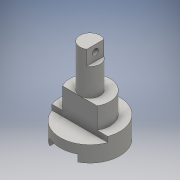
# Autodesk Inventor part: 240628_final4
Saved by Autodesk Inventor 2016 (Build 200138000, 138)
## iProperties
Created: 2024-06-28
Part Number: 240628_final4
Material: 일반
Document SubType Name: Modeling
Designer: pc
Density: 1 g/cm^3
Appearance: 기본값
Author: pc
Autodesk Inventor part; units mm, degrees
ref_plane "YZ Plane" through (0, 0, 0) normal (1, 0, 0) x (0, 1, 0)
ref_plane "XZ Plane" through (0, 0, 0) normal (0, 1, 0) x (-1, 0, 0)
ref_plane "XY Plane" through (0, 0, 0) normal (0, 0, 1) x (1, 0, 0)
sketch "스케치1" plane through (0, 0, 0) normal (0, 0, 1) x (1, 0, 0)
  circle A0 centre (0, 0) radius 14.0239
  constraints: 1 centre point, 1 coincident
extrude "돌출1" add sketch "스케치1" along normal blind 10
sketch "스케치2" plane through (0, 0, 10) normal (0, 0, 1) x (1, 0, 0)
  circle A0 centre (0, 0) radius 9.454
  constraints: 1 centre point, 1 coincident
extrude "돌출2" add sketch "스케치2" along normal blind 10
sketch "스케치3" plane through (0, 0, 20) normal (0, 0, 1) x (1, 0, 0)
  circle A0 centre (0, 0) radius 4.783
  constraints: 1 centre point, 1 coincident
extrude "돌출3" add sketch "스케치3" along normal blind 20
sketch "스케치4" plane through (0, 0, 40) normal (0, 0, 1) x (1, 0, 0)
  circle A0 centre (0, 0) radius 4.783 projected
  line L0 (7.0161, -4.0466) -> (2.5499, -4.0466)
  line L1 (2.5499, -4.0466) -> (2.5499, 4.0466)
  line L2 (2.5499, 4.0466) -> (7.0161, 4.0466)
  line L3 (7.0161, 4.0466) -> (7.0161, -4.0466)
  circle A1 centre (0, 0) radius 4.783 projected
  line L4 (7.0161, -4.0466) -> (2.5499, 4.0466) construction
  line L5 (2.5499, -4.0466) -> (7.0161, 4.0466) construction
  point P0 (4.783, 0)
  constraints: 12 end point, 2 midpoint, 2 parallel, 1 horizontal, 1 horizontal alignment, 1 perpendicular, 3 other
extrude "돌출4" cut sketch "스케치4" against normal blind 7 contours A0 L1 | A0 L2 L3 L0 picked at (3.2943, 0)
sketch "스케치5" plane through (2.5499, -4.0466, 40) normal (1, 0, 0) x (0, 0, -1)
  circle A0 centre (3.1932, 4.0466) radius 1.4587
  point P0 (40, 4.0466)
  constraints: 1 centre point
extrude "돌출5" cut sketch "스케치5" against normal blind 7
sketch "스케치6" plane through (0, 0, 20) normal (0, 0, 1) x (1, 0, 0)
  circle A0 centre (0, 0) radius 14.0239 projected
  line L0 (13.1762, -23.246) -> (-13.1762, -23.246)
  line L1 (-13.1762, -23.246) -> (-13.1762, -4.8019)
  line L2 (-13.1762, -4.8019) -> (13.1762, -4.8019)
  line L3 (13.1762, -4.8019) -> (13.1762, -23.246)
  line L4 (13.1762, -23.246) -> (-13.1762, -4.8019) construction
  line L5 (-13.1762, -23.246) -> (13.1762, -4.8019) construction
  point P0 (0, -14.0239)
  constraints: 12 end point, 2 midpoint, 2 parallel, 2 point on circle, 1 horizontal, 1 perpendicular
extrude "돌출6" cut sketch "스케치6" against normal blind 12.5 contours L2 A0 | A0 L3 L0 L1 picked at (-1.1305, -9.7665)
sketch "스케치7" plane through (0, 0, 0) normal (0, 0, -1) x (-1, 0, 0)
  line L0 (6.585, 15.6352) -> (-6.585, 15.6352)
  line L1 (-6.585, 15.6352) -> (-6.585, -15.6352)
  line L2 (-6.585, -15.6352) -> (6.585, -15.6352)
  line L3 (6.585, -15.6352) -> (6.585, 15.6352)
  line L4 (6.585, 15.6352) -> (-6.585, -15.6352) construction
  line L5 (-6.585, 15.6352) -> (6.585, -15.6352) construction
  point P0 (0, 0)
  constraints: 12 end point, 2 midpoint, 2 parallel, 1 horizontal, 1 perpendicular
extrude "돌출7" cut sketch "스케치7" against normal blind 3.25
